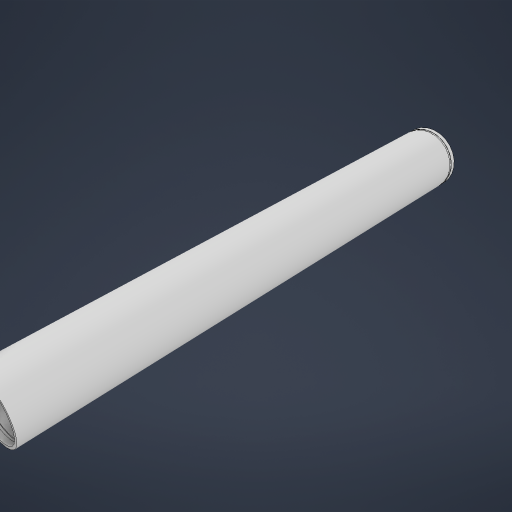
# Autodesk Inventor part: SRM 2020 Casing EE5
Saved by Autodesk Inventor 2024.1 (Build 281209000, 209)
## iProperties
Created: 2023-02-11
Part Number: SRM 2020 Casing EE5
Material: Aluminum 6061
Document SubType Name: Modeling
Designer: Sven
Density: 2.7 g/cm^3
Appearance: Default
Author: Sven
Autodesk Inventor part; units mm, degrees
ref_plane "YZ Plane" through (0, 0, 0) normal (1, 0, 0) x (0, 1, 0)
sketch "Sketch1" plane through (0, 0, 0) normal (0, 0, 1) x (1, 0, 0)
  circle A0 centre (0, 0) radius 24
  circle A1 centre (0, 0) radius 22
  dimension "d0" = 48
  dimension "d1" = 44
  constraints: 2 centre point, 2 coincident
  measures "d0" diameter of A0
  measures "d1" diameter of A1
extrude "Extrusion1" add sketch "Sketch1" along normal blind 384
ref_plane "Work Plane1" through (0, 0, 192) normal (0, 0, 1) x (1, 0, 0)
ref_plane "Work Plane2" through (0, 0, 3.8) normal (0, 0, -1) x (-1, 0, 0)
sketch "Sketch2" plane through (0, 0, 0) normal (0, 0, -1) x (-1, 0, 0)
  circle A0 centre (0, 0) radius 23.25
  circle A1 centre (0, 0) radius 22 projected
  dimension "d4" = 46.5
  constraints: 1 centre point, 1 coincident
  measures "d4" diameter of A0
extrude "Extrusion2" cut sketch "Sketch2" against normal blind 1.85 from surface at -3.8
mirror "Mirror1" about plane through (0, 0, 192) normal (0, 0, 1) of "Extrusion2"
sketch "Sketch3" plane through (0, 0, 0) normal (0, 0, -1) x (-1, 0, 0)
  circle A0 centre (0, 0) radius 23.75
  circle A1 centre (0, 0) radius 24 projected
  dimension "d8" = 47.5
  constraints: 1 centre point, 1 coincident
  measures "d8" diameter of A0
extrude "Extrusion3" cut sketch "Sketch3" against normal up to surface (1.85 mm away) from surface at -3.8
body "Solid2"
